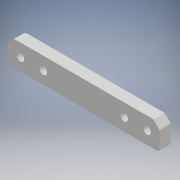
# Autodesk Inventor part: fan_duct_holder
Saved by Autodesk Inventor 2018 (Build 220112000, 112)
## iProperties
Created: 2018-08-16
Part Number: fan_duct_holder
Material: Generic
Document SubType Name: Modeling
Designer: Z. Deniz
Density: 1 g/cm^3
Appearance: Default
Author: Z. Deniz
Autodesk Inventor part; units mm, degrees
ref_plane "YZ Plane" through (0, 0, 0) normal (1, 0, 0) x (0, 1, 0)
ref_plane "XZ Plane" through (0, 0, 0) normal (0, 1, 0) x (-1, 0, 0)
ref_plane "XY Plane" through (0, 0, 0) normal (0, 0, 1) x (1, 0, 0)
sketch "Sketch1" plane through (0, 0, 0) normal (0, 1, 0) x (-1, 0, 0)
  line L0 (0, 0) -> (-60, 0)
  line L1 (-60, 0) -> (-60, -10)
  line L2 (-60, -10) -> (0, -10)
  line L3 (0, -10) -> (0, 0)
  circle A0 centre (-5, -5) radius 1.5
  circle A1 centre (-55, -5) radius 1.5
  line L4 (-30, -10) -> (-30, 0) construction
  line L5 (0, -5) -> (-5, -5) construction
  line L6 (-5, -5) -> (-30, -5) construction
  line L7 (-55, -5) -> (-60, -5) construction
  circle A2 centre (-14, -5) radius 1.5
  line L8 (-30, -5) -> (-55, -5) construction
  circle A3 centre (-46, -5) radius 1.5
  dimension "d0" = 60
  dimension "d1" = 10
  dimension "d2" = 3
  dimension "d3" = 3
  dimension "d4" = 5
  dimension "d5" = 5
  dimension "d6" = 5
  dimension "d7" = 5
  dimension "d9" = 3
  dimension "d10" = 16
  constraints: 18 end point, 5 midpoint, 4 centre point, 2 parallel, 1 horizontal, 1 perpendicular, 1 point on line, 1 symmetric about line, 1 other
  measures "d0" distance of L2.end L1.end
  measures "d1" distance of L1.end L0.end
  measures "d2" diameter of A0
  measures "d3" diameter of A1
  measures "d4" distance from line of L3 L5.end
  measures "d5" distance from line of L1 L7.start
  measures "d6" distance from line of L0 L5.end
  measures "d7" distance from line of L0 L7.start
  measures "d9" diameter of A2
  measures "d10" distance from line of A2.centre L4
extrude "Extrusion1" add sketch "Sketch1" along normal blind 5
chamfer "Chamfer1" distance 2.5 angle 45 2 edges at (0, 2.5, 0) (60, 2.5, 0)
fillet "Fillet1" radius 1 12 edges at (30, 5, 0) (1.25, 5, -1.25) (0, 5, -6.25) (0, 2.5, -2.5) (2.5, 2.5, 0) (57.5, 2.5, 0) (58.75, 5, -1.25) (60, 2.5, -2.5) (60, 5, -6.25) (60, 2.5, -10) (0, 2.5, -10) (30, 5, -10)
equation "\"d3\" = d2"
equation "\"d5\" = d4"
equation "\"d6\" = 0.5 * d1"
equation "\"d7\" = d6"
equation "\"d9\" = d2"
body "Solid1"
